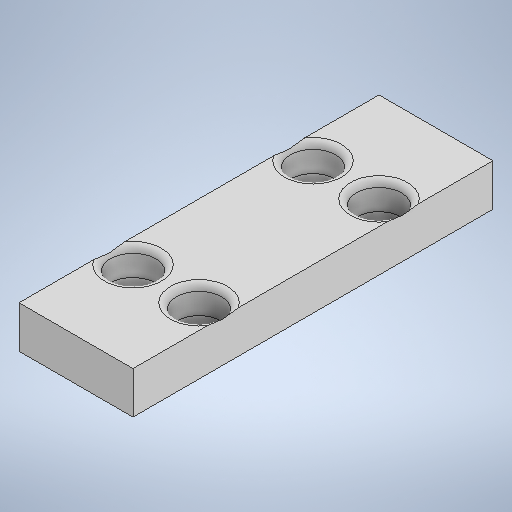
# Autodesk Inventor part: attache_cadre
Saved by Autodesk Inventor 2025.1 (Build 291241000, 241)
## iProperties
Created: 2025-05-14
Part Number: attache_cadre
Material: Générique
Document SubType Name: Modeling
Designer: chapuzet
Density: 1 g/cm^3
Appearance: Par défaut
Author: chapuzet
Autodesk Inventor part; units mm, degrees
ref_plane "YZ Plane" through (0, 0, 0) normal (1, 0, 0) x (0, 1, 0)
ref_plane "XZ Plane" through (0, 0, 0) normal (0, 1, 0) x (-1, 0, 0)
ref_plane "XY Plane" through (0, 0, 0) normal (0, 0, 1) x (1, 0, 0)
sketch "Esquisse1" plane through (0, 0, 0) normal (0, 1, 0) x (-1, 0, 0)
  line L0 (-9.5, 30) -> (9.5, 30)
  line L1 (9.5, 30) -> (9.5, -30)
  line L2 (9.5, -30) -> (-9.5, -30)
  line L3 (-9.5, -30) -> (-9.5, 30)
  line L4 (-9.5, 30) -> (9.5, -30) construction
  line L5 (9.5, 30) -> (-9.5, -30) construction
  circle A0 centre (5.5, 15) radius 1.75
  circle A1 centre (5.5, -15) radius 1.75
  line L6 (0, 32.5338) -> (0, -37.7206)
  circle A2 centre (-5.5, 15) radius 1.75
  circle A3 centre (-5.5, -15) radius 1.75
  point P0 (0, 0)
  dimension "d0" = 19
  dimension "d1" = 60
  dimension "d2" = 15
  dimension "d3" = 15
  dimension "d4" = 3.5
  dimension "d11" = 4
  dimension "d12" = 4
  constraints: 14 end point, 4 centre point, 2 midpoint, 2 parallel, 2 symmetric about line, 1 equal radius, 1 horizontal, 1 perpendicular, 1 vertical, 2 other
  measures "d0" distance of L1.end L2.end
  measures "d1" distance of L0.end L1.end
  measures "d2" distance from line of L0 A0.centre
  measures "d3" distance from line of L2 A1.centre
  measures "d4" diameter of A1
  measures "d11" distance from line of L1 A0.centre
  measures "d12" distance from line of L1 A1.centre
extrude "Extrusion1" add sketch "Esquisse1" along normal blind 7
sketch "Esquisse2" plane through (0, 7, 0) normal (0, 1, 0) x (1, 0, 0)
  circle A0 centre (-5.5, -15) radius 1.75 projected
  circle A1 centre (-5.5, -15) radius 3.75
  circle A2 centre (-5.5, 15) radius 1.75 projected
  circle A3 centre (-5.5, 15) radius 3.75
  line L0 (0, -33.1726) -> (0, 42.5186)
  circle A4 centre (5.5, -15) radius 1.75
  circle A5 centre (5.5, -15) radius 3.75
  circle A6 centre (5.5, 15) radius 1.75
  circle A7 centre (5.5, 15) radius 3.75
  point P0 (0, 0)
  dimension "d7" = 7.5
  constraints: 6 centre point, 4 coincident, 4 symmetric about line, 2 end point, 1 equal radius, 1 vertical, 4 other
  measures "d7" diameter of A3
extrude "Extrusion2" cut sketch "Esquisse2" against normal blind 4.5 contours A1 | A3 | A5 | A6 | A7
fillet "Congé2" radius 1 4 edges at (-9.25, 7, -15) (1.75, 7, -15) (-9.25, 7, 15) (1.75, 7, 15)
